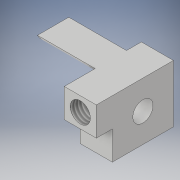
# Autodesk Inventor part: end peice for slides
Saved by Autodesk Inventor 2019 (Build 230136000, 136)
## iProperties
Created: 2019-05-04
Part Number: end peice for slides
Material: Generic
Document SubType Name: Modeling
Designer: User
Density: 1 g/cm^3
Appearance: Default
Author: User
Autodesk Inventor part; units mm, degrees
ref_plane "YZ Plane" through (0, 0, 0) normal (1, 0, 0) x (0, 1, 0)
ref_plane "XZ Plane" through (0, 0, 0) normal (0, 1, 0) x (-1, 0, 0)
ref_plane "XY Plane" through (0, 0, 0) normal (0, 0, 1) x (1, 0, 0)
sketch "Sketch1" plane through (0, 0, 0) normal (1, 0, 0) x (0, 1, 0)
  line L0 (0, 0) -> (11.4, 0)
  line L1 (11.4, 0) -> (11.4, -12.1)
  line L2 (11.4, -12.1) -> (0, -12.1)
  line L3 (0, -12.1) -> (0, 0)
  arc A0 (11.4, -2.9512) -> (11.4, -9.1488) centre (12.8006, -6.05) ccw
  point P0 (3.5, -5)
  dimension "d0" = 11.4
  dimension "d1" = 12.1
  dimension "d2" = 6.1976
  dimension "d3" = 2.9512
  dimension "d29" = 2
  constraints: 8 end point, 2 parallel, 2 point on circle, 2 point on line, 1 centre point, 1 horizontal, 1 perpendicular
  measures "d0" distance of L1.end L2.end
  measures "d1" distance of L0.end L1.end
  measures "d2" distance of A0.end A0.start
  measures "d3" distance of L1.end A0.end
  measures "d29" distance edge to line of A0 L1
extrude "Extrusion1" add sketch "Sketch1" along normal blind 6.35
extrude "Extrusion2" add sketch "Sketch1" against normal blind 11.43 contours L1 A0
sketch "Sketch3" plane through (0, 0, 0) normal (-1, 0, 0) x (0, 0, 1)
  line L0 (0, 11.4) -> (0, 0) projected
  line L1 (0, 0) -> (-12.1, 0) projected
  point P0 (-6.05, 5.7)
  dimension "d19" = 12.1
  dimension "d20" = 6.05
  dimension "d30" = 11.4
  dimension "d31" = 5.7
  measures "d19" distance of L0.end L1.end
  measures "d20" distance from line of L0 point (-6.05, 5.7)
  measures "d30" distance of L0.start L0.end
  measures "d31" distance from line of L1 point (-6.05, 5.7)
sketch "Sketch6" plane through (0, 0, 0) normal (0, 0, 1) x (1, 0, 0)
  line L0 (6.35, 5.7) -> (0, 5.7)
  line L1 (0, 0) -> (0, 11.4) projected
  line L2 (6.35, 11.4) -> (6.35, 0) projected
  line L3 (0, 0) -> (6.35, 0) projected
  line L4 (0, 11.4) -> (6.35, 11.4) projected
  dimension "d33" = 11.4
  dimension "d46" = 5.7
  constraints: 2 end point, 1 horizontal, 1 midpoint
  measures "d33" distance of L2.start L2.end
  measures "d46" distance between parallel lines of L0 L4
hole "Hole2" at (0, 5.7, -6.05) direction (1, 0, 0) diameter 4 end through all
extrude "Extrusion8" add sketch "Sketch6" along normal blind 3.175 contours L0 L1 L4 L2
sketch "Sketch7" plane through (0, 0, 3.175) normal (0, 0, 1) x (1, 0, 0)
  line L0 (6.35, 11.4) -> (0, 11.4) projected
  line L1 (6.35, 5.7) -> (6.35, 11.4) projected
  point P0 (0, 0)
  point P1 (3.175, 8.55)
  dimension "d50" = 6.35
  dimension "d51" = 5.7
  dimension "d52" = 2.85
  dimension "d53" = 3.175
  measures "d50" distance of L0.start L0.end
  measures "d51" distance of L1.start L0.start
  measures "d52" distance from line of point (3.175, 8.55) L0
  measures "d53" distance from line of L1 point (3.175, 8.55)
sketch "Sketch8" plane through (0, 0, 3.175) normal (0, 0, 1) x (1, 0, 0)
  circle A0 centre (3.175, 8.55) radius 2
  line L0 (6.35, 11.4) -> (0, 11.4) projected
  line L1 (6.35, 5.7) -> (6.35, 11.4) projected
  point P0 (0, 0)
  dimension "d63" = 2.85
  dimension "d64" = 3.175
  dimension "d65" = 4
  constraints: 1 centre point
  measures "d63" distance from line of L0 A0.centre
  measures "d64" distance from line of L1 A0.centre
  measures "d65" diameter of A0
extrude "Extrusion9" cut sketch "Sketch8" against normal up to surface (3.175 mm away)
thread "Thread2" size "M4x0.7" class "6H" standard "ISO Metric profile" full length
equation "\"d3\" = -0.5 * d2 + 0.5 * d1"
equation "\"d20\" = 0.5 * d19"
equation "\"d31\" = 0.5 * d30"
equation "\"d46\" = 0.5 * d33"
equation "\"d52\" = 0.5 * d51"
equation "\"d53\" = 0.5 * d50"
equation "\"d63\" = d52"
equation "\"d64\" = d53"
body "Solid1"
